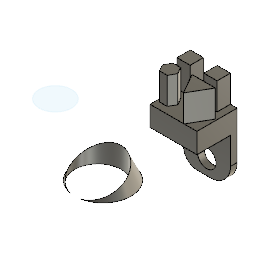
Chair v1 (Autodesk Fusion 360 design; units mm, degrees)
Autodesk Fusion 360 part; units mm, degrees
sketch "Sketch2" plane through (0, 0, 0) normal (0, 0, 1) x (1, 0, 0)
  circle A0 centre (-7.0427, -3.2785) radius 38.0087
  line L0 (36.4391, -77.432) -> (-44.4308, -77.432)
  dimension "d1" = 10
extrude "Extrude1" add sketch "Sketch2" along normal blind 30 draft -25 makes body 1
sketch "Sketch3" plane through (0, 0, 30) normal (0, 0, 1) x (-1, 0, 0)
  circle A0 centre (7.0427, 3.2785) radius 24.0195
sketch "Sketch4" plane through (0, 0, 30) normal (0, 0, 1) x (-1, 0, 0)
  line L0 (-70, -120) -> (-90, -120)
  line L1 (-90, -120) -> (-90, -100)
  line L2 (-90, -100) -> (-70, -100)
  line L3 (-70, -100) -> (-70, -120)
  line L4 (-110, -120) -> (-130, -120)
  line L5 (-130, -120) -> (-130, -100)
  line L6 (-130, -100) -> (-110, -100)
  line L7 (-110, -100) -> (-110, -120)
  line L8 (-85.7735, -70) -> (-91.547, -80)
  line L9 (-91.547, -80) -> (-85.7735, -90)
  line L10 (-85.7735, -90) -> (-74.2265, -90)
  line L11 (-74.2265, -90) -> (-68.453, -80)
  line L12 (-68.453, -80) -> (-74.2265, -70)
  line L13 (-74.2265, -70) -> (-85.7735, -70)
  line L14 (-103.2678, -89.4547) -> (-120.5883, -59.4547)
  line L15 (-120.5883, -59.4547) -> (-137.9088, -89.4547)
  line L16 (-137.9088, -89.4547) -> (-103.2678, -89.4547)
  point P0 (-80, -80)
  point P1 (-120.5883, -79.4547)
  constraint horizontal L0
  constraint vertical L1
  constraint horizontal L2
  constraint vertical L3
  constraint horizontal L4
  constraint vertical L5
  constraint horizontal L6
  constraint vertical L7
extrude "Extrude2" add sketch "Sketch4" along normal blind 40 separate body makes body 2 at (116.6667, 120, 43.3333) makes body 3 at (70.3775, 76.6667, 43.3333) makes body 4 at (76.6667, 120, 43.3333) makes body 5 at (126.3618, 69.4547, 43.3333)
sketch "Sketch5" plane through (0, 0, 0) normal (0, 0, 1) x (1, 0, 0)
  line L0 (70, 120) -> (140, 120)
  line L1 (140, 120) -> (140, 60)
  line L2 (140, 60) -> (70, 60)
  line L3 (70, 60) -> (70, 120)
  constraint horizontal L0
  constraint vertical L1
  constraint horizontal L2
  constraint vertical L3
extrude "Extrude3" add sketch "Sketch5" along normal blind 30 bodies 2 3 4 5
sketch "Sketch8" plane through (0, 0, 0) normal (0, 0, -1) x (1, 0, 0)
  line L0 (140, -60) -> (70, -60)
  line L1 (70, -60) -> (70, -120)
  line L2 (70, -120) -> (140, -120)
  line L3 (140, -120) -> (140, -60)
  line L4 (140, -120) -> (70, -120)
  line L5 (70, -120) -> (70, -110)
  line L6 (70, -110) -> (140, -110)
  line L7 (140, -110) -> (140, -120)
  constraint horizontal L4
  constraint vertical L5
  constraint horizontal L6
  constraint vertical L7
  constraint coincident L2.end L3.start
extrude "Extrude4" add sketch "Sketch8" along normal blind 70 contours L1 L2 L3 L4 L5 L6 L7 bodies 2
fillet "Fillet1" radius 20 1 edges at (70, 115, -70) on bodies 2
fillet "Fillet2" radius 30 1 edges at (140, 115, -70) on bodies 2
sketch "Sketch9" plane through (0, 110, 0) normal (0, -1, 0) x (1, 0, 0)
  arc A0 (110, -70) -> (140, -40) centre (110, -40) ccw
  line L0 (140, -40) -> (140, 0)
  line L1 (140, 0) -> (70, 0)
  line L2 (70, 0) -> (70, -50)
  arc A1 (70, -50) -> (90, -70) centre (90, -50) ccw
  line L3 (90, -70) -> (110, -70)
  circle A2 centre (104.5172, -47.1352) radius 13.5251
extrude "Extrude5" cut sketch "Sketch9" against normal blind 70 contours A2 bodies 2
move_body "Move1" bodies 1 to x (1, 0, 0) y (0, 1, 0) z (0, 0, 1) at (60, 0, -50)
sketch "Sketch10" plane through (0, 0, -50) normal (0, 0, -1) x (1, 0, 0)
  circle A0 centre (52.9573, 3.2785) radius 38.0087
  circle A1 centre (52.9573, 0) radius 34.503
extrude "Extrude6" cut sketch "Sketch10" against normal blind 60 contours A1 bodies 1
move_face "MoveFace1" to x (1, 0, 0) y (0, 1, 0) z (0, 0, 1) at (0, 10.673, 8.0747) 1 faces at (81.4345, -24.8868, -45.1503) on bodies 1
